z_top_fix_1.2 (Autodesk Fusion 360 design; units mm, degrees)
Autodesk Fusion 360 part; units mm, degrees
sketch "base_top_holes" plane through (0, 0, 0) normal (0, 0, 1) x (1, 0, 0)
  line L0 (0, 0) -> (38, 0)
  line L1 (38, 0) -> (38, 33)
  line L2 (8, 45) -> (0, 45)
  line L3 (0, 45) -> (0, 0)
  line L4 (8, 45) -> (8, 0)
  line L5 (8, 4.01) -> (30.5, 4.01)
  circle A0 centre (29.3, 8) radius 4.05
  circle A1 centre (16, 15) radius 7.7 construction
  circle A2 centre (16, 33) radius 8 construction
  circle A3 centre (29.3, 25) radius 5.75
  line L6 (16, 15) -> (16, 33) construction
  line L7 (29.3, 8) -> (29.3, 25) construction
  line L8 (20, 39.9282) -> (12, 39.9282)
  line L9 (12, 39.9282) -> (8, 33)
  line L10 (8, 33) -> (12, 26.0718)
  line L11 (12, 26.0718) -> (20, 26.0718)
  line L12 (20, 26.0718) -> (24, 33)
  line L13 (24, 33) -> (20, 39.9282)
  line L14 (23.7, 15) -> (19.85, 21.6684)
  line L15 (19.85, 21.6684) -> (12.15, 21.6684)
  line L16 (12.15, 21.6684) -> (8.3, 15)
  line L17 (8.3, 15) -> (12.15, 8.3316)
  line L18 (12.15, 8.3316) -> (19.85, 8.3316)
  line L19 (19.85, 8.3316) -> (23.7, 15)
  line L20 (28.3, 23) -> (30.3, 23)
  line L21 (30.3, 23) -> (30.3, 8)
  line L22 (30.3, 8) -> (28.3, 8)
  line L23 (28.3, 8) -> (28.3, 23)
  line L24 (30.5, 4.01) -> (30.5, 0)
  circle A4 centre (29.3, 8) radius 2.55
  line L25 (38, 33) -> (8, 33)
  line L26 (4, 0) -> (4, 45)
  point P0 (16, 33)
  point P1 (16, 15)
  dimension "d1" = 38
  dimension "d2" = 45
  dimension "d3" = 8
  dimension "d5" = 8.1
  dimension "d6" = 29.3
  dimension "d7" = 8
  dimension "d8" = 16
  dimension "d9" = 15
  dimension "d10" = 33
  dimension "d11" = 25
  dimension "d12" = 16
  dimension "d13" = 15.4
  dimension "d14" = 11.5
  dimension "d15" = 15
  dimension "d16" = 2
  dimension "d17" = 4.01
  dimension "d18" = 7.5
  dimension "d41" = 1.5
  measures "d1" distance of L0.start L0.end
  measures "d2" distance of L0.start L2.end
  measures "d3" distance of L2.end L2.start
  measures "d5" diameter of A0
  measures "d6" distance of L3 A0.centre
  measures "d7" distance of L0.start A0.centre
  measures "d8" distance of L0.start P1
  measures "d9" distance of L0.start P1
  measures "d10" distance of L0.start A2.centre
  measures "d11" distance of L0.start A3.centre
  measures "d12" diameter of A2
  measures "d13" diameter of A1
  measures "d14" diameter of A3
  measures "d15" distance of L20.end L21.end
  measures "d16" distance of L21.end L22.end
  measures "d17" distance of L5.end L24.end
  measures "d18" distance of L1 L24
  measures "d41" distance of A0 A4
extrude "Extrude1" add sketch "base_top_holes" against normal blind 6.5 contours L0 L2 L3 L26 | L0 L2 L4 L26 | L0 L4 L5 A0 L24 | L0 L1 L4 L5 A0 A3 L10 L11 L12 L21 L23 L24 L25 makes body 1
extrude "Extrude2" add sketch "base_top_holes" along normal blind 11 contours L0 L2 L3 L26 bodies 1
extrude "Extrude3" add sketch "base_top_holes" along normal blind 7 contours L0 L2 L4 L26 | L0 L4 L5 A0 L24 bodies 1
extrude "Extrude7" add sketch "base_top_holes" along normal blind 2 from surface at -6.5 contours L5 A0 L21 L23 A4 | L5 A0 bodies 1
sketch "frame_holes" plane through (0, 0, 0) normal (-1, 0, 0) x (0, -1, 0)
  line L0 (-45, 11) -> (-45, -6.5)
  line L1 (-45, -6.5) -> (0, -6.5)
  line L2 (0, -6.5) -> (0, 11)
  line L3 (0, 11) -> (-45, 11)
  line L4 (0, -6.5) -> (-45, -6.5)
  line L5 (0, -6.5) -> (0, 11)
  circle A0 centre (-15, 5) radius 3.1
  circle A1 centre (-35, 5) radius 3.1
  circle A2 centre (-35, 5) radius 1.75
  circle A3 centre (-15, 5) radius 1.75
  line L6 (-35, 5) -> (-15, 5) construction
  line L7 (0, 7) -> (-45, 7)
  line L8 (0, 7) -> (-45, 7)
  line L9 (-45, 7) -> (-45, 11)
  line L10 (-45, 11) -> (0, 11)
  line L11 (0, 11) -> (0, 7)
  line L12 (-38.1, 7) -> (-38.1, 5)
  line L13 (-31.9, 5) -> (-31.9, 7)
  line L14 (-18.1, 5) -> (-18.1, 7)
  line L15 (-11.9, 5) -> (-11.9, 7)
  dimension "d26" = 3.5
  dimension "d27" = 3.5
  dimension "d28" = 15
  dimension "d29" = 20
  dimension "d30" = 11.5
  dimension "d31" = 6.2
  dimension "d32" = 6.2
  measures "d26" diameter of A2
  measures "d27" diameter of A3
  measures "d28" distance of L1.end A0.centre
  measures "d29" distance of A0.centre A1.centre
  measures "d30" distance of L1.end A0.centre
  measures "d31" diameter of A1
  measures "d32" diameter of A0
extrude "Extrude5" cut sketch "frame_holes" against normal up to surface (8 mm away) contours A1 L7 L8 L12 | A1 L7 L8 | A1 L7 L8 | A0 L7 L8 L15 | A1 L7 L8 L13 | A0 L7 L8 | A0 L7 L8 | A0 L7 L8 L14 | A2 | A3 bodies 1
extrude "Extrude6" add sketch "frame_holes" against normal blind 4 contours A1 L7 L8 L12 | A1 L7 L8 | A1 L7 L8 | A0 L7 L8 L15 | A1 L7 L8 L13 | A0 L7 L8 | A0 L7 L8 | A0 L7 L8 L14 bodies 1
chamfer "Chamfer1" distance 2 angle 45 4 edges at (8, 7.955, 7) (8, 25, 7) (8, 41.55, 7) (4, 22.5, 11) on bodies 1
chamfer "Chamfer2" distance 7 angle 45 1 edges at (30.5, 2.005, 7) on bodies 1
chamfer "Chamfer3" distance 5 angle 45 2 edges at (38, 33, -3.25) (38, 0, -3.25) on bodies 1
chamfer "Chamfer4" distance 5.8 angle 45 1 edges at (8, 45, -0.75) on bodies 1
sketch "chamfer_line" plane through (0, 0, 0) normal (-1, 0, 0) x (0, -1, 0)
  circle A0 centre (-35, 5) radius 1.75
  circle A1 centre (-15, 5) radius 1.75
  line L0 (-45, 11) -> (-45, -6.5)
  line L1 (-45, -6.5) -> (0, -6.5)
  line L2 (0, -6.5) -> (0, 11)
  line L3 (0, 11) -> (-45, 11)
  line L4 (0, -6.5) -> (0, 11)
  line L5 (0, -6.5) -> (-45, -6.5)
  line L6 (-11.5, -6.5) -> (0, 5)
  dimension "d58" = 11.5
  dimension "d59" = 11.5
  measures "d58" distance of L1.end L6.start
  measures "d59" distance of L1.end L6.end
ref_plane "WorkPlane1" through (0, 5.75, -0.75) normal (-0.707107, 0.5, 0.5) x (0, -0.707107, 0.707107)
sketch "chamfer" plane through (0, 5.75, -0.75) normal (-0.707107, 0.5, 0.5) x (0, -0.707107, 0.707107)
  line L0 (0, -5.75) -> (12.3744, 3)
  line L1 (0, -5.75) -> (-31.8198, 16.75)
  line L2 (-8.1317, 0) -> (8.1317, 0)
  point P0 (8.1317, 0)
extrude "Extrude8" cut sketch "chamfer" against normal blind 30 bodies 1
sketch "rod_reinforcement" plane through (0, 0, 0) normal (0, 0, 1) x (-1, 0, 0)
  line L0 (-33, 0) -> (-38, -5)
  line L1 (-38, -5) -> (-38, -28)
  line L2 (-38, -28) -> (-33, -33)
  line L3 (-33, -33) -> (-24, -33)
  line L4 (-24, -33) -> (-20, -26.0718)
  line L5 (-20, -26.0718) -> (-12, -26.0718)
  line L6 (-12, -26.0718) -> (-8, -33)
  line L7 (-8, -33) -> (-8, -4.01)
  line L8 (-8.3, -15) -> (-12.15, -21.6684)
  line L9 (-12.15, -21.6684) -> (-19.85, -21.6684)
  line L10 (-19.85, -21.6684) -> (-23.7, -15)
  line L11 (-23.7, -15) -> (-19.85, -8.3316)
  line L12 (-19.85, -8.3316) -> (-12.15, -8.3316)
  line L13 (-12.15, -8.3316) -> (-8.3, -15)
  line L14 (-8, -4.01) -> (-28.6054, -4.01)
  arc A0 (-28.3, -11.9246) -> (-28.6054, -4.01) centre (-29.3, -8) ccw
  line L15 (-28.3, -11.9246) -> (-28.3, -19.3376)
  arc A1 (-30.3, -19.3376) -> (-28.3, -19.3376) centre (-29.3, -25) ccw
  line L16 (-30.3, -19.3376) -> (-30.3, -11.9246)
  arc A2 (-29.9946, -4.01) -> (-30.3, -11.9246) centre (-29.3, -8) ccw
  line L17 (-29.9946, -4.01) -> (-30.5, -4.01)
  line L18 (-30.5, -4.01) -> (-30.5, 0)
  line L19 (-30.5, 0) -> (-33, 0)
  arc A3 (-30.3, -19.3376) -> (-28.3, -19.3376) centre (-29.3, -25) ccw
  arc A4 (-28.3, -10.3457) -> (-30.3, -10.3457) centre (-29.3, -8) ccw
  circle A5 centre (-29.3, -25) radius 12.5 construction
  line L20 (-29.3, -25) -> (-20.4612, -16.1612)
  line L21 (-38, -5) -> (-38, -28)
  circle A6 centre (-22.4057, -18.1057) radius 2.75 construction
  circle A7 centre (-22.4057, -18.1057) radius 3.1
  circle A8 centre (-29.3, -8) radius 6
  line L22 (-30.3, -19.3376) -> (-30.3, -11.9246)
  line L23 (-28.3, -11.9246) -> (-28.3, -19.3376)
  arc A9 (-28.3, -11.9246) -> (-28.6054, -4.01) centre (-29.3, -8) ccw
  arc A10 (-29.9946, -4.01) -> (-30.3, -11.9246) centre (-29.3, -8) ccw
  arc A11 (-28.6054, -4.01) -> (-29.9946, -4.01) centre (-29.3, -8) ccw
  dimension "d72" = 25
  dimension "d73" = 45
  dimension "d74" = 5.5
  dimension "d75" = 6.2
  dimension "d76" = 12
  measures "d72" diameter of A5
  measures "d73" angle of L1 L20
  measures "d74" diameter of A6
  measures "d75" diameter of A7
  measures "d76" diameter of A8
extrude "Extrude11" add sketch "rod_reinforcement" along normal blind 2 contours L14 L17 L18 A8 A11 | L16 A2 L17 L18 A8 L22 A10 | L14 A0 L15 A8 L23 A9 bodies 1
chamfer "Chamfer6" distance 5 angle 45 1 edges at (0, 0, 8) on bodies 1
chamfer "Chamfer9" distance 1.5 angle 45 1 edges at (0, 28.25, -6.5) on bodies 1
chamfer "Chamfer10" distance 0.26 distance2 3 6 edges at (10.225, 18.3342, -6.5) (10.225, 11.6658, -6.5) (16, 8.3316, -6.5) (21.775, 11.6658, -6.5) (21.775, 18.3342, -6.5) (16, 21.6684, -6.5) measured on face at (3.6667, 29.1262, -6.5) measured on face at (3.6667, 29.1262, -6.5) measured on face at (3.6667, 29.1262, -6.5) measured on face at (3.6667, 29.1262, -6.5) measured on face at (3.6667, 29.1262, -6.5) measured on face at (3.6667, 29.1262, -6.5) on bodies 1
mirror "Mirror2" about plane through (0, 0, 0) normal (0, 1, 0) of bodies 1 makes body 2
move_body "Move2" bodies 2 to x (1, 0, 0) y (0, 1, 0) z (0, 0, 1) at (0, -3, 0)
equation "d27 = d26"
equation "d32 = d31"
named bodies: "z_top_fix_right", "z_top_fix_left"
